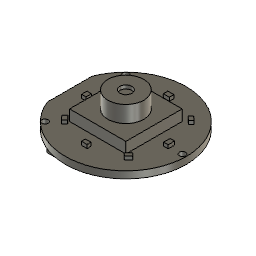
Case (Autodesk Fusion 360 archive; units mm, degrees)
design "qr-scanner-GM861XS"
Autodesk Fusion 360 part; units mm, degrees
sketch "Sketch1" plane through (0, 0, 0) normal (0, 0, 1) x (1, 0, 0)
  line L0 (-7.9924, 3.1752) -> (-7.9924, -3.1752)
  arc A0 (-7.9924, -3.1752) -> (-7.9924, 3.1752) centre (0, 0) ccw
  dimension "d1" = 17.2
  constraint coincident A0.centre origin
  constraint vertical L0
  measures "d1" diameter of A0
extrude "Extrude1" add sketch "Sketch1" along normal blind 1
sketch "Sketch2" plane through (0, 0, 1) normal (0, 0, 1) x (-1, 0, 0)
  line L0 (4, 4) -> (-4, 4)
  line L1 (-4, 4) -> (-4, -4)
  line L2 (-4, -4) -> (4, -4)
  line L3 (4, -4) -> (4, 4)
  arc A0 (7.9924, 3.1752) -> (7.9924, -3.1752) centre (0, 0) ccw
  line L4 (7.9924, -3.1752) -> (7.9924, 3.1752)
  point P0 (-4, 0)
  point P1 (0, 4)
  dimension "d4" = 8
  dimension "d5" = 8
  constraint horizontal L0
  constraint vertical L1
  constraint horizontal L2
  constraint vertical L3
  constraint midpoint L1 P0
  constraint midpoint L0 P1
  constraint vertical P1 A0.centre
  constraint horizontal P0 A0.centre
  constraint coincident A0.centre origin
  measures "d4" distance of L0.start L2.end
  measures "d5" distance of L1.end L2.end
extrude "Extrude2" add sketch "Sketch2" along normal blind 1.55 contours L0 L1 L2 L3
sketch "Sketch3" plane through (0, 0, 2.55) normal (0, 0, 1) x (-1, 0, 0)
  line L0 (4, -4) -> (4, 4)
  line L1 (4, 4) -> (-4, 4)
  line L2 (-4, 4) -> (-4, -4)
  line L3 (-4, -4) -> (4, -4)
  circle A0 centre (0, 0) radius 2.5612
  constraint coincident A0.centre origin
extrude "Extrude3" add sketch "Sketch3" along normal blind 2.35 contours A0
sketch "Sketch4" plane through (0, 0, 0) normal (0, 0, -1) x (1, 0, 0)
  line L0 (-7.0133, 4.25) -> (-4.5133, 4.25)
  line L1 (-4.5133, 4.25) -> (-4.5133, -4.25)
  line L2 (-4.5133, -4.25) -> (-7.0133, -4.25)
  line L3 (-7.0133, -4.25) -> (-7.0133, 4.25)
  arc A0 (-7.9924, -3.1752) -> (-7.9924, 3.1752) centre (0, 0) ccw
  line L4 (-7.9924, 3.1752) -> (-7.9924, -3.1752)
  point P0 (-5.7633, 4.25)
  point P1 (-7.0133, 0)
  dimension "d10" = 2.5
  dimension "d11" = 8.5
  constraint horizontal L0
  constraint vertical L1
  constraint horizontal L2
  constraint vertical L3
  constraint midpoint L0 P0
  constraint midpoint L3 P1
  measures "d10" distance of L0.start L0.end
  measures "d11" distance of L0.start L2.end
extrude "Extrude4" add sketch "Sketch4" along normal blind 4.2 contours L0 L1 L2 L3
sketch "Sketch5" plane through (0, 0, 1) normal (0, 0, 1) x (-1, 0, 0)
  line L0 (4, -4) -> (-4, -4)
  line L1 (-4, -4) -> (-4, 4)
  line L2 (-4, 4) -> (4, 4)
  line L3 (4, 4) -> (4, -4)
  circle A0 centre (5.7366, 5.7566) radius 0.45
  circle A1 centre (5.7712, -5.7516) radius 0.45
  circle A2 centre (-8.0266, -0.0192) radius 0.45
  arc A3 (7.9924, 3.1752) -> (7.9924, -3.1752) centre (0, 0) ccw
  line L4 (7.9924, -3.1752) -> (7.9924, 3.1752)
  dimension "d14" = 0.9
  dimension "d15" = 0.9
  dimension "d16" = 0.9
  measures "d14" diameter of A0
  measures "d15" diameter of A1
  measures "d16" diameter of A2
hole "Hole1" at (-5.7366, -5.7566, 1) at (-5.7712, 5.7516, 1) at (8.0266, 0.0192, 1) direction (0, 0, -1) diameter 0.9 end through all
sketch "Sketch6" plane through (0, 0, 4.9) normal (0, 0, 1) x (-1, 0, 0)
  circle A0 centre (0, 0) radius 2.5612
  circle A1 centre (0, 0) radius 0.8574
  constraint concentric A0 A1
extrude "Extrude5" cut sketch "Sketch6" against normal blind 0.5 contours A1
sketch "Sketch7" plane through (0, 0, 0) normal (0, 0, -1) x (1, 0, 0)
  circle A0 centre (-5.7712, -5.7516) radius 0.45
  circle A1 centre (-5.7366, 5.7566) radius 0.45
  circle A2 centre (8.0266, -0.0192) radius 0.45
  line L0 (-7.0133, -4.25) -> (-7.0133, 4.25)
  line L1 (-7.0133, 4.25) -> (-4.5133, 4.25)
  line L2 (-4.5133, 4.25) -> (-4.5133, -4.25)
  line L3 (-4.5133, -4.25) -> (-7.0133, -4.25)
  arc A3 (-7.9924, -3.1752) -> (-7.9924, 3.1752) centre (0, 0) ccw
  line L4 (-7.9924, 3.1752) -> (-7.9924, -3.1752)
  line L5 (-4.2403, -6.0832) -> (-3.2403, -6.0832)
  line L6 (-3.2403, -6.0832) -> (-3.2403, -5.5832)
  line L7 (-3.2403, -5.5832) -> (-4.2403, -5.5832)
  line L8 (-4.2403, -5.5832) -> (-4.2403, -6.0832)
  line L9 (-2.2599, -6.8555) -> (-1.2599, -6.8555)
  line L10 (-1.2599, -6.8555) -> (-1.2599, -4.8555)
  line L11 (-1.2599, -4.8555) -> (-2.2599, -4.8555)
  line L12 (-2.2599, -4.8555) -> (-2.2599, -6.8555)
  dimension "d21" = 1
  dimension "d22" = 0.5
  dimension "d23" = 1
  dimension "d24" = 2
  constraint horizontal L5
  constraint vertical L6
  constraint horizontal L7
  constraint vertical L8
  constraint horizontal L9
  constraint vertical L10
  constraint horizontal L11
  constraint vertical L12
  measures "d21" distance of L5.start L5.end
  measures "d22" distance of L5.start L7.end
  measures "d23" distance of L9.start L9.end
  measures "d24" distance of L9.start L11.end
extrude "Extrude6" add sketch "Sketch7" along normal blind 1 contours L5 L6 L7 L8 | L9 L10 L11 L12
sketch "Sketch8" plane through (0, 0, 1) normal (0, 0, 1) x (-1, 0, 0)
  circle A0 centre (5.7712, -5.7516) radius 0.45
  circle A1 centre (5.7366, 5.7566) radius 0.45
  circle A2 centre (-8.0266, -0.0192) radius 0.45
  line L0 (4, -4) -> (-4, -4)
  line L1 (-4, -4) -> (-4, 4)
  line L2 (-4, 4) -> (4, 4)
  line L3 (4, 4) -> (4, -4)
  arc A3 (7.9924, 3.1752) -> (7.9924, -3.1752) centre (0, 0) ccw
  line L4 (7.9924, -3.1752) -> (7.9924, 3.1752)
  line L5 (0.2182, 6.091) -> (-0.5813, 6.091)
  line L6 (-0.5813, 6.091) -> (-0.5813, 5.5267)
  line L7 (-0.5813, 5.5267) -> (0.2182, 5.5267)
  line L8 (0.2182, 5.5267) -> (0.2182, 6.091)
  line L9 (5.991, 0.3073) -> (5.364, 0.3073)
  line L10 (5.364, 0.3073) -> (5.364, -0.4766)
  line L11 (5.364, -0.4766) -> (5.991, -0.4766)
  line L12 (5.991, -0.4766) -> (5.991, 0.3073)
  line L13 (0.2653, -5.5821) -> (-0.6126, -5.5821)
  line L14 (-0.6126, -5.5821) -> (-0.6126, -6.2248)
  line L15 (-0.6126, -6.2248) -> (0.2653, -6.2248)
  line L16 (0.2653, -6.2248) -> (0.2653, -5.5821)
  line L17 (-5.7244, 0.3642) -> (-6.3671, 0.3642)
  line L18 (-6.3671, 0.3642) -> (-6.3671, -0.5607)
  line L19 (-6.3671, -0.5607) -> (-5.7244, -0.5607)
  line L20 (-5.7244, -0.5607) -> (-5.7244, 0.3642)
  line L21 (-4.82, -4.0739) -> (-5.2049, -4.4745)
  line L22 (-5.2049, -4.4745) -> (-4.6576, -5.0004)
  line L23 (-4.6576, -5.0004) -> (-4.2727, -4.5997)
  line L24 (-4.2727, -4.5997) -> (-4.82, -4.0739)
  line L25 (-4.6173, 4.852) -> (-5.232, 4.25)
  line L26 (-5.232, 4.25) -> (-4.8446, 3.8543)
  line L27 (-4.8446, 3.8543) -> (-4.2298, 4.4563)
  line L28 (-4.2298, 4.4563) -> (-4.6173, 4.852)
  line L29 (4.2775, 4.8826) -> (3.8201, 4.4628)
  line L30 (3.8201, 4.4628) -> (4.3704, 3.8634)
  line L31 (4.3704, 3.8634) -> (4.8277, 4.2831)
  line L32 (4.8277, 4.2831) -> (4.2775, 4.8826)
  line L33 (4.7584, -4.636) -> (4.3697, -4.2471)
  line L34 (4.3697, -4.2471) -> (3.8011, -4.8154)
  line L35 (3.8011, -4.8154) -> (4.1898, -5.2043)
  line L36 (4.1898, -5.2043) -> (4.7584, -4.636)
  constraint horizontal L5
  constraint vertical L6
  constraint horizontal L7
  constraint vertical L8
  constraint horizontal L9
  constraint vertical L10
  constraint horizontal L11
  constraint vertical L12
  constraint horizontal L13
  constraint vertical L14
  constraint horizontal L15
  constraint vertical L16
  constraint horizontal L17
  constraint vertical L18
  constraint horizontal L19
  constraint vertical L20
  constraint perpendicular L21 L22
  constraint perpendicular L22 L23
  constraint equal L22 L24
  constraint equal L21 L23
  constraint perpendicular L25 L26
  constraint perpendicular L26 L27
  constraint equal L26 L28
  constraint equal L25 L27
  constraint perpendicular L29 L32
  constraint equal L30 L32
  constraint equal L29 L31
  constraint perpendicular L33 L34
  constraint perpendicular L34 L35
  constraint equal L34 L36
  constraint equal L33 L35
extrude "Extrude7" add sketch "Sketch8" along normal blind 0.5 contours L5 L6 L7 L8 | L9 L10 L11 L12 | L13 L14 L15 L16 | L17 L18 L19 L20 | L21 L22 L23 L24 | L25 L26 L27 L28 | L29 L30 L31 L32 | L33 L34 L35 L36
equation "d8 = 3.9 mm - 1.55 mm"

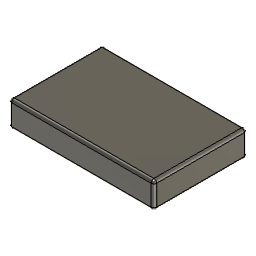
design "RS PRO, 3.7 V, Lithium Polymer Rechargeable Battery, 1.8 Ah"
Autodesk Fusion 360 part; units mm, degrees
sketch "Sketch1" plane through (0, 0, 0) normal (0, 0, 1) x (1, 0, 0)
  line L0 (-28.0455, 17.5284) -> (23.8545, 17.5284)
  line L1 (23.8545, 17.5284) -> (23.8545, -15.8716)
  line L2 (23.8545, -15.8716) -> (-28.0455, -15.8716)
  line L3 (-28.0455, -15.8716) -> (-28.0455, 17.5284)
  dimension "d1" = 51.9
  dimension "d2" = 33.4
  constraint horizontal L0
  constraint vertical L1
  constraint horizontal L2
  constraint vertical L3
  measures "d1" distance of L0.start L0.end
  measures "d2" distance of L0.end L1.end
extrude "Extrude1" add sketch "Sketch1" along normal blind 9.4
sketch "Sketch2" plane through (0, 0, 9.4) normal (0, 0, 1) x (-1, 0, 0)
  line L0 (28.0455, 15.8716) -> (-23.8545, 15.8716)
  line L1 (-23.8545, 15.8716) -> (-23.8545, -17.5284)
  line L2 (-23.8545, -17.5284) -> (28.0455, -17.5284)
  line L3 (28.0455, -17.5284) -> (28.0455, 15.8716)
  line L4 (27.9621, 16.0005) -> (-23.8545, 15.8716) construction
  line L5 (-23.8545, 15.8716) -> (-23.7711, -17.6573) construction
  line L6 (-23.7711, -17.6573) -> (28.0455, -17.5284) construction
  line L7 (28.0455, -17.5284) -> (27.9621, 16.0005) construction
  dimension "d5" = 10
  constraint coincident L2.end
  constraint coincident L0.end
extrude "Extrude2" [suppressed]
fillet "Fillet1" radius 1 6 faces at (-10.7455, -4.7383, 9.4) (6.5545, -15.8716, 3.1333) (-28.0455, -4.7383, 3.1333) (-10.7455, 17.5284, 3.1333) (23.8545, 6.3951, 3.1333) (-10.7455, -4.7383, 0)
equation "d6 = 'Battery'"
